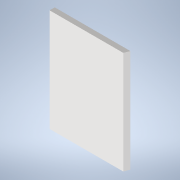
# Autodesk Inventor part: PlatteInnenEineSeite
Saved by Autodesk Inventor 2020.3 (Build 243373010, 373A)
## iProperties
Created: 2021-02-11
Part Number: PlatteInnenEineSeite
Material: Generisch
Document SubType Name: Modeling
Designer: Stefan
Density: 1 g/cm^3
Appearance: Vorgabe
Author: Stefan
Autodesk Inventor part; units mm, degrees
ref_plane "YZ Plane" through (0, 0, 0) normal (1, 0, 0) x (0, 1, 0)
ref_plane "XZ Plane" through (0, 0, 0) normal (0, 1, 0) x (-1, 0, 0)
ref_plane "XY Plane" through (0, 0, 0) normal (0, 0, 1) x (1, 0, 0)
sketch "Skizze1" plane through (0, 0, 0) normal (0, 0, 1) x (1, 0, 0)
  line L0 (-147.195, 0) -> (0, 0)
  line L1 (0, 0) -> (0, -200)
  line L2 (0, -200) -> (-147.195, -200)
  line L3 (-147.195, -200) -> (-147.195, 0)
  point P0 (0, 0)
  dimension "d0" = 147.195
  dimension "d1" = 200
  dimension "d2" = 0
  dimension "d3" = 0
  constraints: 8 end point, 2 parallel, 1 horizontal, 1 perpendicular
  measures "d0" distance of L1.end L2.end
  measures "d1" distance of L0.end L1.end
  measures "d2" distance from line of point (0, 0) L1
  measures "d3" distance from line of point (0, 0) L0
extrude "Extrusion1" add sketch "Skizze1" along normal blind 10
sketch "Skizze2" plane through (-147.195, 0, 0) normal (0, 1, 0) x (1, 0, 0)
  line L0 (0, -10) -> (147.195, -10) projected
  line L1 (0, 0) -> (147.195, 0) projected
  line L2 (147.195, -10) -> (147.195, 0)
  line L3 (147.195, -10) -> (143.37, -10)
  line L4 (143.37, -10) -> (147.195, 0)
  dimension "d6" = 3.825
  dimension "d7" = 110.932
  constraints: 6 end point, 1 point on line, 1 vertical
  measures "d6" distance of L0.end L3.end
  measures "d7" angle of L0 L4
extrude "Extrusion2" cut sketch "Skizze2" against normal through all
